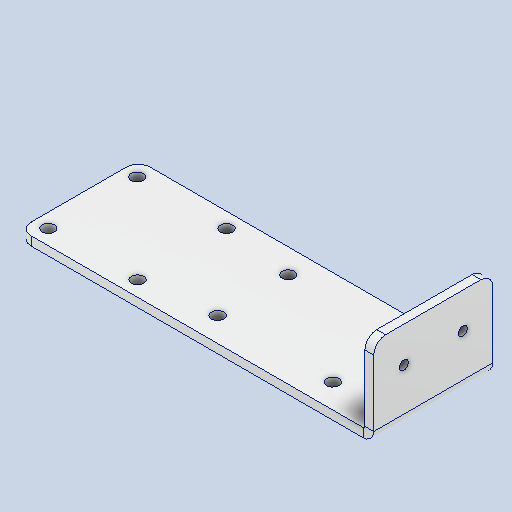
# Autodesk Inventor part: servo-horn_bottom
Saved by Autodesk Inventor 2023 (Build 270158000, 158)
## iProperties
Created: 2022-10-09
Part Number: servo-horn_bottom
Material: 알루미늄 6061
Document SubType Name: Sheet Metal
Designer: 박동준
Density: 2.7 g/cm^3
Sheet Metal Rule: Default_mm
Appearance: 알루미늄 - 평지
Flat Pattern Width: 2.014 cm
Flat Pattern Length: 7.22793 cm
Flat Pattern Area: 14.557 cm^2
Sheet Metal Width: 20.140 mm
Sheet Metal Length: 72.279 mm
Sheet Metal Area: 1455.705 mm^2
품번: 18
Author: 박동준
Autodesk Inventor part; units mm, degrees
ref_plane "YZ Plane" through (0, 0, 0) normal (1, 0, 0) x (0, 1, 0)
ref_plane "XZ Plane" through (0, 0, 0) normal (0, 1, 0) x (-1, 0, 0)
ref_plane "XY Plane" through (0, 0, 0) normal (0, 0, 1) x (1, 0, 0)
sketch "스케치1" plane through (0, 0, 0) normal (0, 1, 0) x (-1, 0, 0)
  line L0 (30, -10.07) -> (-30, -10.07)
  line L1 (-30, -10.07) -> (-30, 10.07)
  line L2 (-30, 10.07) -> (30, 10.07)
  line L3 (30, 10.07) -> (30, -10.07)
  point P0 (0, 0)
  point P1 (0, -10.07)
  point P2 (30, 0)
  dimension "d0" = 20.14
  dimension "d1" = 60
  measures "d0" distance between parallel lines of L2 L0
  measures "d1" distance of L0.start L0.end
extrude "판1" add sketch "스케치1" along normal mid plane 1.5
sketch "스케치2" plane through (28.5, -0.75, -10.07) normal (1, 0, 0) x (0, 1, 0)
  line L0 (0, 20.14) -> (0, 0)
  line L1 (0, 0) -> (15, 0)
  line L2 (15, 0) -> (15, 20.14)
  line L3 (15, 20.14) -> (0, 20.14)
  constraints: 6 end point, 1 horizontal, 1 perpendicular, 1 vertical
edge flange "플랜지1" height 15 angle 90 thickness 1.5 bend radius 0.31 thickness toward (1, 0, 0) relief tear relief width 1.5 relief depth 0.75 edges at (30, 0.75, 0) wall of the first edge with corners at (28.5, -0.75, 10.07) (28.5, -0.75, -10.07) (28.5, 14.25, -10.07) (28.5, 14.25, 10.07)
bend "절곡부1"
corner "구석1"
sketch "스케치3" plane through (0, 0.75, 0) normal (0, 1, 0) x (1, 0, 0)
  line L0 (-30, -10.07) -> (-30, 10.07) projected
  line L1 (-27.62, 7.525) -> (-27.62, -7.525) construction
  circle A0 centre (-27.62, 7.525) radius 1.05
  circle A1 centre (-27.62, -7.525) radius 1.05
  line L2 (-12.52, 7.525) -> (-12.52, -7.525) construction
  circle A2 centre (-12.52, 7.525) radius 1.05
  circle A3 centre (-12.52, -7.525) radius 1.05
  point P0 (0, 0)
  point P1 (-27.62, 0)
  point P2 (-12.52, 0)
  dimension "d14" = 2.38
  dimension "d15" = 2.38
  dimension "d16" = 15.05
  dimension "d18" = 2.1
  dimension "d20" = 2.1
  dimension "d30" = 15.1
  dimension "d31" = 15.05
  dimension "d32" = 2.1
  dimension "d33" = 2.1
  constraints: 4 centre point, 4 coincident, 4 end point, 2 horizontal alignment, 2 midpoint, 1 vertical
  measures "d14" distance from line of L0 L1.start
  measures "d15" distance from line of L0 L1.end
  measures "d16" distance of L1.end L1.start
  measures "d18" diameter of A0
  measures "d20" diameter of A1
  measures "d30" distance of L2.start A0.centre
  measures "d31" distance of L2.end L2.start
  measures "d32" diameter of A2
  measures "d33" diameter of A3
extrude "돌출1" cut sketch "스케치3" against normal through all
sketch "스케치4" plane through (30, 14.25, 10.07) normal (1, 0, 0) x (0, 0, -1)
  line L0 (0, 0) -> (20.14, 0) projected
  line L1 (5.07, -6) -> (15.07, -6) construction
  point P0 (10.07, -14.25)
  point P1 (10.07, 0)
  point P2 (10.07, 0)
  point P3 (10.07, 0)
  point P4 (10.07, -6)
  dimension "d34" = 6
  dimension "d38" = 10
  constraints: 4 midpoint, 3 horizontal alignment, 2 coincident, 2 end point, 1 horizontal, 1 vertical alignment
  measures "d34" distance from line of L0 L1.end
  measures "d38" distance of L1.end L1.start
fillet "모깎기1" radius 2 4 edges at (29.25, 14.25, 10.07) (29.25, 14.25, -10.07) (-30, 0, 10.07) (-30, 0, -10.07)
hole "구멍1" at (30, 8.25, 5) at (30, 8.25, -5) direction (-1, 0, 0) diameter 1.567 end through all thread size "M2x0.4" class "6H" standard "ISO Metric profile"
sketch "Sketch5" plane through (0, -0.75, 0) normal (0, -1, 0) x (1, 0, 0)
  circle A0 centre (-27.62, 7.525) radius 1.05 projected
  circle A1 centre (-12.52, 7.525) radius 1.05 projected
  circle A2 centre (-27.62, -7.525) radius 1.05 projected
  circle A3 centre (-12.52, -7.525) radius 1.05 projected
  arc A4 (-30, -8.07) -> (-28, -10.07) centre (-28, -8.07) ccw projected
  line L0 (-28, -10.07) -> (28.19, -10.07) projected
  line L1 (28.19, -10.07) -> (28.19, 10.07) projected
  line L2 (28.19, 10.07) -> (-28, 10.07) projected
  arc A5 (-28, 10.07) -> (-30, 8.07) centre (-28, 8.07) ccw projected
  line L3 (-30, 8.07) -> (-30, -8.07) projected
  line L4 (-30, 0) -> (28.19, 0) construction
  circle A6 centre (-0.52, -5.975) radius 0.7835 projected
  circle A7 centre (18.98, -5.975) radius 0.7835 projected
  circle A8 centre (-0.52, -5.975) radius 1.05
  circle A9 centre (18.98, -5.975) radius 1.05
  circle A10 centre (-0.52, 5.975) radius 1.05
  circle A11 centre (18.98, 5.975) radius 1.05
  point P0 (0, 0)
  dimension "d46" = 2.1
  constraints: 4 centre point, 2 coincident, 2 end point, 2 midpoint, 2 symmetric about line, 1 equal radius, 2 other
  measures "d46" diameter of A8
extrude "Cut1" cut sketch "Sketch5" against normal blind 1.5 contours A6 | A7 | A8 | A9 | A10 | A11
equation "\"d3\" = BendReliefWidth"
equation "\"d4\" = BendReliefDepth"
equation "\"d5\" = MinimumRemnant"
equation "\"d6\" = TransitionRadius"
equation "\"d10\" = CornerReliefSize"
equation "\"TransitionRadius\" = BendRadius"
equation "\"BendReliefWidth\" = 1.5"
equation "\"BendReliefDepth\" = 0.75"
equation "\"MinimumRemnant\" = 3"
equation "\"CornerReliefSize\" = 6"
equation "\"BendRadius\" = 0.31"
